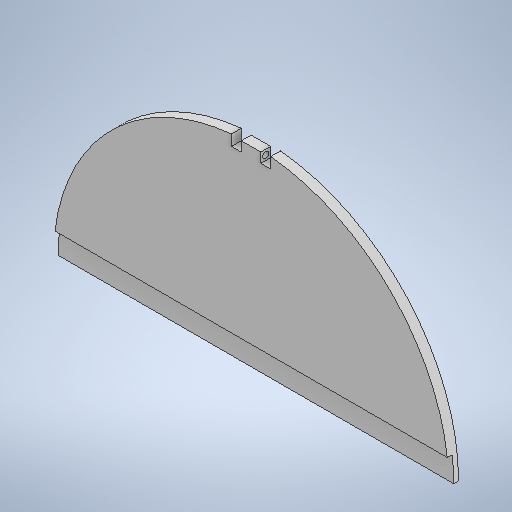
# Autodesk Inventor part: Flap
Saved by Autodesk Inventor 2025.2 (Build 292293000, 293)
## iProperties
Created: 2025-06-02
Part Number: Flap
Material: Generic
Document SubType Name: Modeling
Designer: dylan
Density: 1 g/cm^3
Appearance: Default
Author: dylan
Autodesk Inventor part; units mm, degrees
ref_plane "YZ Plane" through (0, 0, 0) normal (1, 0, 0) x (0, 1, 0)
ref_plane "XZ Plane" through (0, 0, 0) normal (0, 1, 0) x (-1, 0, 0)
ref_plane "XY Plane" through (0, 0, 0) normal (0, 0, 1) x (1, 0, 0)
sketch "Sketch4" plane through (0, 0, 0) normal (0, 0, 1) x (1, 0, 0)
  circle A0 centre (0, 0) radius 505
  line L0 (0, 0) -> (0, 505)
  line L1 (0, 505) -> (0, 500)
  line L2 (0, 500) -> (25, 500)
  line L3 (0, 500) -> (-25, 500)
  line L4 (-25, 500) -> (-25, 450)
  line L5 (25, 500) -> (25, 450)
  line L6 (25, 450) -> (50, 450)
  line L7 (50, 450) -> (50, 502.5187)
  line L8 (-25, 450) -> (-50, 450)
  line L9 (-50, 450) -> (-50, 502.5187)
  line L10 (505, 0) -> (-505, 0)
  line L11 (-505, 0) -> (505, 0)
  line L12 (505, 0) -> (505, 62.2415)
  line L13 (505, 62.2415) -> (-505, 62.2415)
  line L14 (-505, 62.2415) -> (-505, 0)
  point P0 (-501.1497, 62.2415)
  point P1 (501.1497, 62.2415)
  dimension "d17" = 1010
  dimension "d18" = 5
  dimension "d19" = 25
  dimension "d20" = 25
  dimension "d22" = 50
  dimension "d23" = 50
  dimension "d24" = 25
  dimension "d25" = 25
  dimension "d36" = 62.2415
  constraints: 30 end point, 6 horizontal, 5 point on circle, 5 vertical, 2 parallel, 1 centre point, 1 coincident, 1 perpendicular, 1 point on line
  measures "d17" diameter of A0
  measures "d18" distance of L0.end L1.end
  measures "d19" distance of L1.end L2.end
  measures "d20" distance of L1.end L3.end
  measures "d22" distance of L3.end L4.end
  measures "d23" distance of L2.end L5.end
  measures "d24" distance of L5.end L6.end
  measures "d25" distance of L4.end L8.end
  measures "d36" distance between parallel lines of L13 L10
extrude "Extrusion4" add sketch "Sketch4" along normal blind 25 contours A0 L13 L0 L2 L5 L6 L7 | L9 L8 L4 L3 L0 L13 A0
sketch "Sketch5" plane through (25, 450, 0) normal (1, 0, 0) x (0, 0, -1)
  line L0 (-25, 0) -> (-25, 50) projected
  line L1 (-25, 50) -> (-12.5, 50) construction
  line L2 (0, 50) -> (-25, 50) projected
  line L3 (-12.5, 50) -> (-12.5, 37.5) construction
  circle A0 centre (-12.5, 37.5) radius 7.9375
  point P0 (0, -450)
  dimension "d28" = 12.5
  dimension "d29" = 15.875
  constraints: 4 end point, 1 centre point, 1 coincident, 1 midpoint, 1 vertical
  measures "d28" distance of L1.end L3.end
  measures "d29" diameter of A0
extrude "Extrusion5" cut sketch "Sketch5" against normal up to surface (50 mm away)
sketch "Sketch6" plane through (-50, 450, 0) normal (0, 1, 0) x (1, 0, 0)
  line L0 (-455, -25) -> (555, -25) projected
  line L1 (0, 0) -> (0, -25) projected
  line L2 (25, -25) -> (0, -25)
  line L3 (0, -25) -> (0, 0)
  line L4 (0, 0) -> (25, 0)
  line L5 (25, 0) -> (25, -25)
  line L6 (75, 0) -> (100, 0)
  line L7 (100, 0) -> (100, -25)
  line L8 (100, -25) -> (75, -25)
  line L9 (75, -25) -> (75, 0)
  point P0 (50, 0)
  constraints: 16 end point, 4 parallel, 3 point on line, 2 horizontal, 2 perpendicular
extrude "Extrusion6" add sketch "Sketch6" along normal blind 25
extrude "Extrusion8" add sketch "Sketch4" along normal blind 12.5 contours A0 L10 L0 L13 | L0 L10 A0 L13
body "Solid2"
